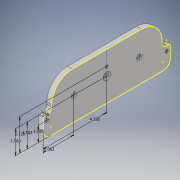
# Autodesk Inventor part: Base plate
Saved by Autodesk Inventor 2017.1 (Build 211199000, 199)
## iProperties
Created: 2017-04-17
Part Number: Base plate
Material: Generic
Document SubType Name: Modeling
Designer: rbibb
Density: 1 g/cm^3
Appearance: Default
Author: rbibb
Autodesk Inventor part; units mm, degrees
ref_plane "YZ Plane" through (0, 0, 0) normal (1, 0, 0) x (0, 1, 0)
ref_plane "XZ Plane" through (0, 0, 0) normal (0, 1, 0) x (-1, 0, 0)
ref_plane "XY Plane" through (0, 0, 0) normal (0, 0, 1) x (1, 0, 0)
sketch "Sketch1" plane through (0, 0, 0) normal (1, 0, 0) x (0, 1, 0)
  line L0 (12.7, 0) -> (33.3375, 0)
  line L1 (33.3375, -215.9) -> (12.7, -215.9)
  line L2 (0, -203.2) -> (0, -12.7)
  line L3 (41.275, -14.2875) -> (44.45, -14.2875)
  line L4 (79.375, -49.2125) -> (79.375, -166.6875)
  line L5 (44.45, -201.6125) -> (41.275, -201.6125)
  line L6 (0, -210.6276) -> (0, -5.2724)
  line L7 (33.3375, 0) -> (33.3375, -6.35)
  line L8 (33.3375, -209.55) -> (33.3375, -215.9)
  arc A0 (79.375, -49.2125) -> (44.45, -14.2875) centre (44.45, -49.2125) ccw
  arc A1 (44.45, -201.6125) -> (79.375, -166.6875) centre (44.45, -166.6875) ccw
  arc A2 (33.3375, -6.35) -> (41.275, -14.2875) centre (41.275, -6.35) ccw
  arc A3 (41.275, -201.6125) -> (33.3375, -209.55) centre (41.275, -209.55) ccw
  arc A4 (12.7, 0) -> (0, -12.7) centre (12.7, -12.7) ccw
  arc A5 (0, -203.2) -> (12.7, -215.9) centre (12.7, -203.2) ccw
  point P0 (0, 0)
  point P1 (0, -215.9)
  point P2 (79.375, -201.6125)
  point P3 (79.375, -107.95)
  point P4 (33.3375, -107.95)
  dimension "d0" = 215.9
  dimension "d1" = 79.375
  dimension "d2" = 33.3375
  dimension "d3" = 14.2875
  dimension "d4" = 14.2875
  dimension "d5" = 34.925
  dimension "d6" = 34.925
  dimension "d7" = 7.9375
  dimension "d8" = 12.7
  dimension "d9" = 12.7
  constraints: 18 end point, 12 point on circle, 12 tangent, 7 point on line, 6 centre point, 5 parallel, 3 perpendicular, 2 horizontal, 1 equal radius, 1 horizontal alignment, 1 midpoint
  measures "d0" distance of point (0, -215.9) point (0, 0)
  measures "d1" horizontal distance of point (79.375, -201.612) point (0, -215.9)
  measures "d2" distance of L1.start point (0, -215.9)
  measures "d3" distance between parallel lines of L3 L0
  measures "d4" distance between parallel lines of L5 L1
  measures "d5" radius of A0
  measures "d6" radius of A1
  measures "d7" radius of A2
  measures "d8" radius of A4
  measures "d9" radius of A5
extrude "Extrusion1" add sketch "Sketch1" along normal blind 7.9375
sketch "Sketch2" plane through (7.9375, 0, 0) normal (1, 0, 0) x (0, 0, -1)
  line L0 (215.9, 12.7) -> (215.9, 33.3375) projected
  line L1 (215.9, 33.3375) -> (209.55, 33.3375) projected
  arc A0 (201.6125, 41.275) -> (209.55, 33.3375) centre (209.55, 41.275) ccw projected
  line L2 (201.6125, 41.275) -> (201.6125, 44.45) projected
  arc A1 (201.6125, 44.45) -> (166.6875, 79.375) centre (166.6875, 44.45) ccw projected
  line L3 (166.6875, 79.375) -> (49.2125, 79.375) projected
  arc A2 (49.2125, 79.375) -> (14.2875, 44.45) centre (49.2125, 44.45) ccw projected
  line L4 (14.2875, 44.45) -> (14.2875, 41.275) projected
  arc A3 (6.35, 33.3375) -> (14.2875, 41.275) centre (6.35, 41.275) ccw projected
  line L5 (6.35, 33.3375) -> (0, 33.3375) projected
  line L6 (0, 33.3375) -> (0, 12.7) projected
  arc A4 (0, 12.7) -> (12.7, 0) centre (12.7, 12.7) ccw projected
  line L7 (12.7, 0) -> (203.2, 0) projected
  arc A5 (203.2, 0) -> (215.9, 12.7) centre (203.2, 12.7) ccw projected
  line L8 (107.95, 79.375) -> (107.95, 0) construction
  point P0 (0, 0)
  point P1 (6.35, 25.4)
  point P2 (52.3875, 39.7002)
  point P3 (107.95, 53.975)
  point P4 (107.95, 39.7002)
  point P5 (209.55, 25.4)
  point P6 (163.5125, 39.7002)
  dimension "d12" = 107.95
  dimension "d13" = 39.7002
  dimension "d15" = 39.7002
  dimension "d16" = 53.975
  dimension "d17" = 52.3875
  dimension "d18" = 6.35
  dimension "d19" = 25.4
  constraints: 2 end point, 2 midpoint, 2 symmetric about line
  measures "d12" distance from line of L6 point (107.95, 39.7)
  measures "d13" distance from line of point (107.95, 39.7) L7
  measures "d15" distance from line of L7 point (52.388, 39.7)
  measures "d16" distance from line of L7 point (107.95, 53.975)
  measures "d17" distance from line of point (52.388, 39.7) L6
  measures "d18" distance from line of L6 point (6.35, 25.4)
  measures "d19" distance from line of L7 point (6.35, 25.4)
sketch "Sketch3" plane through (7.9375, 0, 0) normal (1, 0, 0) x (0, 0, -1)
  line L0 (49.2125, 79.375) -> (166.6875, 79.375) construction
  line L1 (107.95, 79.375) -> (107.95, 0) construction
  point P0 (0, 0)
  constraints: 2 end point, 1 midpoint, 1 vertical
hole "Hole1" at (7.9375, 39.7002, -107.95) direction (-1, 0, 0) diameter 12.7 depth 25.4 tip angle 118
hole "Hole2" at (7.9375, 53.975, -107.95) direction (-1, 0, 0) diameter 4.9784 depth 25.4 tip angle 118 thread size "1/4-20 UNC" class "2B" standard "ANSI Unified Screw Threads"
hole "Hole3" at (7.9375, 25.4, -6.35) at (7.9375, 25.4, -209.55) direction (-1, 0, 0) diameter 4.9784 depth 25.4 tip angle 118 thread size "1/4-20 UNC" class "2B" standard "ANSI Unified Screw Threads"
hole "Hole4" at (7.9375, 39.7002, -52.3875) at (7.9375, 39.7002, -163.5125) direction (-1, 0, 0) diameter 6.35 depth 25.4 tip angle 118 countersink diameter 9.525 countersink angle 86
body "Solid1"
